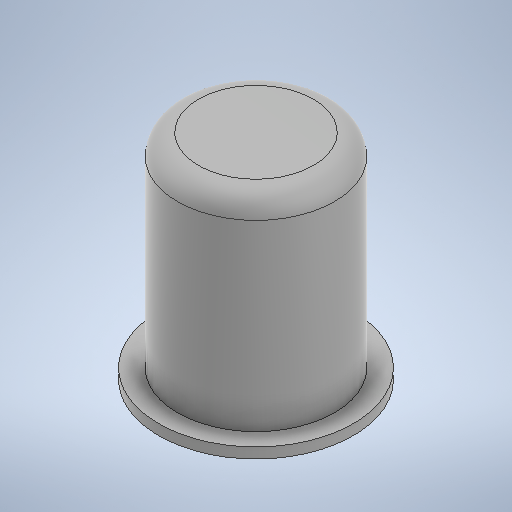
# Autodesk Inventor part: Knob
Saved by Autodesk Inventor 2025 (Build 290162010, 162A)
## iProperties
Created: 2025-09-13
Part Number: Knob
Material: Genérico
Document SubType Name: Modeling
Designer: João Vitor
Density: 1 g/cm^3
Appearance: Padrão
Author: João Vitor
Autodesk Inventor part; units mm, degrees
ref_plane "YZ Plane" through (0, 0, 0) normal (1, 0, 0) x (0, 1, 0)
ref_plane "XZ Plane" through (0, 0, 0) normal (0, 1, 0) x (-1, 0, 0)
ref_plane "XY Plane" through (0, 0, 0) normal (0, 0, 1) x (1, 0, 0)
sketch "Esboço1" plane through (0, 0, 0) normal (0, 1, 0) x (-1, 0, 0)
  circle A0 centre (0, 0) radius 9.3
  dimension "d0" = 18.6
  constraints: 1 centre point, 1 coincident
  measures "d0" diameter of A0
extrude "Extrusão1" add sketch "Esboço1" along normal blind 1
sketch "Esboço2" plane through (0, 1, 0) normal (0, 1, 0) x (1, 0, 0)
  circle A0 centre (0, 0) radius 8.3
  circle A1 centre (0, 0) radius 9.3 projected
  circle A2 centre (0, 0) radius 7.5
  dimension "d3" = 1
  dimension "d4" = 15
  constraints: 2 centre point, 2 coincident
  measures "d3" radial gap between concentric circles of A1 A0
  measures "d4" diameter of A2
extrude "Extrusão2" add sketch "Esboço2" along normal blind 19.5 contours A2
fillet "Arredondamento1" radius 2 1 edges at (-7.5, 20.5, 0)
sketch "Esboço6" plane through (0, 0, 0) normal (0, -1, 0) x (1, 0, 0)
  circle A0 centre (0, 0) radius 3.25
  dimension "d13" = 6.5
  constraints: 1 centre point, 1 coincident
  measures "d13" diameter of A0
extrude "Extrusão5" cut sketch "Esboço6" against normal blind 10
